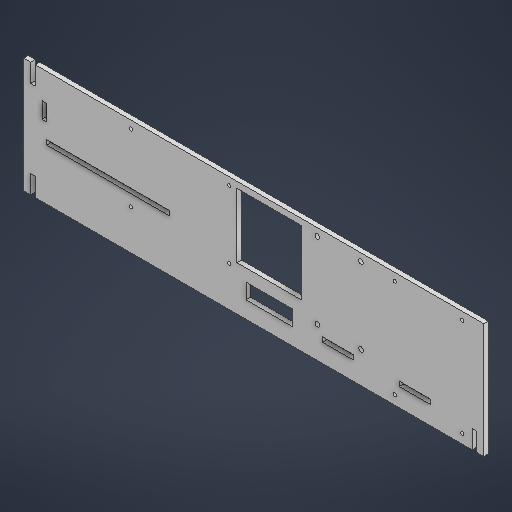
# Autodesk Inventor part: 2ndSideboard
Saved by Autodesk Inventor 2027 (Build 310192000, 192)
## iProperties
Created: 2026-06-01
Part Number: 2ndSideboard
Material: Generic
Document SubType Name: Modeling
Designer: alexy
Density: 1 g/cm^3
Appearance: Default
Author: alexy
Autodesk Inventor part; units mm, degrees
ref_plane "YZ Plane" through (0, 0, 0) normal (1, 0, 0) x (0, 1, 0)
ref_plane "XZ Plane" through (0, 0, 0) normal (0, 1, 0) x (-1, 0, 0)
ref_plane "XY Plane" through (0, 0, 0) normal (0, 0, 1) x (1, 0, 0)
sketch "Sketch1" plane through (0, 0, 0) normal (0, 0, 1) x (1, 0, 0)
  line L0 (0, 0) -> (300, 0)
  line L1 (300, 0) -> (300, 65)
  line L2 (300, 65) -> (0, 65)
  line L3 (0, 65) -> (0, 0)
  line L4 (0, 0) -> (300, 0)
  line L5 (300, 0) -> (300, -10)
  line L6 (300, -10) -> (0, -10)
  line L7 (0, -10) -> (0, 0)
  dimension "d0" = 300
  dimension "d1" = 65
  dimension "d2" = 10
  constraints: 16 end point, 4 parallel, 2 horizontal, 2 perpendicular, 1 vertical alignment
  measures "d0" distance of L1.end L2.end
  measures "d1" distance of L0.end L1.end
  measures "d2" distance of L4.end L5.end
extrude "Extrusion1" add sketch "Sketch1" along normal blind 3
sketch "Sketch3" plane through (0, 0, 3) normal (0, 0, 1) x (1, 0, 0)
  line L0 (139, 61) -> (181, 61)
  line L1 (181, 61) -> (181, 19)
  line L2 (181, 19) -> (139, 19)
  line L3 (139, 19) -> (139, 61)
  line L4 (139, 61) -> (181, 19) construction
  line L5 (181, 61) -> (139, 19) construction
  line L6 (300, -10) -> (300, 65) projected
  line L7 (300, 65) -> (0, 65) projected
  line L8 (0, 65) -> (0, -10) projected
  line L9 (145, 11) -> (175, 11)
  line L10 (175, 11) -> (175, 1)
  line L11 (175, 1) -> (145, 1)
  line L12 (145, 1) -> (145, 11)
  line L13 (145, 11) -> (175, 1) construction
  line L14 (175, 11) -> (145, 1) construction
  point P0 (0, 0)
  point P1 (160, 40)
  point P2 (160, 6)
  dimension "d12" = 25
  dimension "d13" = 42
  dimension "d14" = 42
  dimension "d19" = 160
  dimension "d57" = 8
  dimension "d58" = 30
  dimension "d59" = 10
  constraints: 24 end point, 4 midpoint, 4 parallel, 2 horizontal, 2 perpendicular, 1 vertical alignment
  measures "d12" distance from line of L7 point (160, 40)
  measures "d13" distance of L0.end L1.end
  measures "d14" distance of L1.end L2.end
  measures "d19" distance from line of L8 point (160, 40)
  measures "d57" distance between parallel lines of L2 L9
  measures "d58" distance of L10.end L11.end
  measures "d59" distance of L9.end L10.end
extrude "Extrusion2" cut sketch "Sketch3" against normal blind 3
sketch "Sketch2" plane through (0, 0, 3) normal (0, 0, 1) x (1, 0, 0)
  line L0 (0, -10) -> (300, -10) projected
  line L1 (4.5, -10) -> (7.5, -10)
  line L2 (7.5, -10) -> (7.5, 2)
  line L3 (7.5, 2) -> (4.5, 2)
  line L4 (4.5, 2) -> (4.5, -10)
  line L5 (295.5, -10) -> (292.5, -10)
  line L6 (292.5, -10) -> (292.5, 2)
  line L7 (292.5, 2) -> (295.5, 2)
  line L8 (295.5, 2) -> (295.5, -10)
  line L9 (300, 65) -> (0, 65) projected
  line L10 (4.5, 65) -> (7.5, 65)
  line L11 (7.5, 65) -> (7.5, 53)
  line L12 (7.5, 53) -> (4.5, 53)
  line L13 (4.5, 53) -> (4.5, 65)
  line L14 (0, 65) -> (0, -10) projected
  point P0 (0, 0)
  point P1 (294, 2)
  dimension "d5" = 4.5
  dimension "d6" = 12
  dimension "d7" = 3
  dimension "d8" = 6
  dimension "d9" = 3
  dimension "d53" = 12
  dimension "d54" = 3
  dimension "d55" = 4.5
  constraints: 24 end point, 6 parallel, 3 horizontal, 3 perpendicular, 3 point on line, 1 horizontal alignment, 1 midpoint
  measures "d5" distance of L0.start L1.start
  measures "d6" distance of L1.end L2.end
  measures "d7" distance of L1.start L1.end
  measures "d8" horizontal distance of L0.end point (294, 2)
  measures "d9" distance between parallel lines of L6 L8
  measures "d53" distance of L10.end L11.end
  measures "d54" distance of L11.end L12.end
  measures "d55" distance between parallel lines of L14 L13
extrude "Extrusion3" cut sketch "Sketch2" against normal blind 3
sketch "Sketch4" plane through (0, 0, 3) normal (0, 0, 1) x (1, 0, 0)
  line L0 (15.05, 26.5) -> (95.15, 26.5)
  line L1 (95.15, 26.5) -> (95.15, 23.45)
  line L2 (95.15, 23.45) -> (15.05, 23.45)
  line L3 (15.05, 23.45) -> (15.05, 26.5)
  line L4 (12, 47) -> (15.05, 47)
  line L5 (15.05, 47) -> (15.05, 36.5)
  line L6 (15.05, 36.5) -> (12, 36.5)
  line L7 (12, 36.5) -> (12, 47)
  line L8 (0, 65) -> (0, -10) projected
  point P0 (0, 0)
  point P1 (139, 19)
  dimension "d20" = 80.1
  dimension "d21" = 3.05
  dimension "d22" = 3.05
  dimension "d23" = 10.5
  dimension "d28" = 12
  dimension "d56" = 18
  dimension "d60" = 10
  constraints: 16 end point, 4 parallel, 2 horizontal, 2 perpendicular, 1 vertical alignment
  measures "d20" distance of L1.end L2.end
  measures "d21" distance of L0.end L1.end
  measures "d22" distance of L4.start L4.end
  measures "d23" distance of L6.end L4.start
  measures "d28" distance from line of L8 L4.start
  measures "d56" vertical distance of L8.start L4.start
  measures "d60" distance of L0.start L5.end
extrude "Extrusion4" cut sketch "Sketch4" against normal blind 3
sketch "Sketch5" plane through (0, 0, 3) normal (0, 0, 1) x (1, 0, 0)
  circle A0 centre (191.5, 60) radius 1.55
  circle A1 centre (220, 60) radius 1.55
  circle A2 centre (220, 10.5) radius 1.55
  circle A3 centre (191.5, 10.5) radius 1.55
  line L0 (300, -10) -> (300, 65) projected
  point P0 (0, 0)
  dimension "d31" = 28.5
  dimension "d32" = 49.5
  dimension "d33" = 3.1
  dimension "d34" = 3.1
  dimension "d35" = 3.1
  dimension "d36" = 3.1
  dimension "d37" = 80
  dimension "d38" = 5
  constraints: 4 centre point, 2 horizontal alignment, 2 vertical alignment
  measures "d31" distance of A1.centre A0.centre
  measures "d32" distance of A2.centre A1.centre
  measures "d33" diameter of A0
  measures "d34" diameter of A1
  measures "d35" diameter of A2
  measures "d36" diameter of A3
  measures "d37" distance from line of L0 A1.centre
  measures "d38" vertical distance of L0.end A1.centre
extrude "Extrusion5" cut sketch "Sketch5" against normal blind 3
sketch "Sketch6" plane through (0, 0, 3) normal (0, 0, 1) x (1, 0, 0)
  circle A0 centre (242, 60) radius 1.1
  circle A1 centre (286, 60) radius 1.1
  circle A2 centre (286, -4) radius 1.1
  circle A3 centre (242, -4) radius 1.1
  circle A4 centre (220, 60) radius 1.55 projected
  circle A5 centre (70, 60) radius 1.1
  circle A6 centre (134, 60) radius 1.1
  circle A7 centre (134, 16) radius 1.1
  circle A8 centre (70, 16) radius 1.1
  point P0 (0, 0)
  point P1 (300, 65)
  point P2 (0, 65)
  dimension "d41" = 2.2
  dimension "d42" = 2.2
  dimension "d43" = 2.2
  dimension "d44" = 2.2
  dimension "d45" = 64
  dimension "d46" = 44
  dimension "d50" = 5
  dimension "d51" = 14
  dimension "d61" = 64
  dimension "d62" = 44
  dimension "d63" = 2.2
  dimension "d64" = 2.2
  dimension "d65" = 2.2
  dimension "d66" = 2.2
  dimension "d67" = 70
  dimension "d68" = 5
  constraints: 8 centre point, 4 horizontal alignment, 4 vertical alignment
  measures "d41" diameter of A0
  measures "d42" diameter of A1
  measures "d43" diameter of A2
  measures "d44" diameter of A3
  measures "d45" distance of A3.centre A0.centre
  measures "d46" distance of A0.centre A1.centre
  measures "d50" vertical distance of point (300, 65) A1.centre
  measures "d51" horizontal distance of point (300, 65) A1.centre
  measures "d61" distance of A5.centre A6.centre
  measures "d62" distance of A7.centre A6.centre
  measures "d63" diameter of A6
  measures "d64" diameter of A7
  measures "d65" diameter of A8
  measures "d66" diameter of A5
  measures "d67" horizontal distance of point (0, 65) A5.centre
  measures "d68" vertical distance of point (0, 65) A5.centre
extrude "Extrusion6" cut sketch "Sketch6" against normal blind 3 contours A0 | A1 | A2 | A3 | A5 | A6 | A7 | A8
sketch "Sketch7" plane through (0, 0, 3) normal (0, 0, 1) x (1, 0, 0)
  line L0 (244.95, 5.05) -> (265, 5.05)
  line L1 (265, 5.05) -> (265, 2)
  line L2 (265, 2) -> (244.95, 2)
  line L3 (244.95, 2) -> (244.95, 5.05)
  line L4 (194.9, 5.05) -> (215, 5.05)
  line L5 (215, 5.05) -> (215, 2)
  line L6 (215, 2) -> (194.9, 2)
  line L7 (194.9, 2) -> (194.9, 5.05)
  line L8 (300, -10) -> (300, 65) projected
  point P0 (0, 0)
  dimension "d69" = 20.05
  dimension "d70" = 3.05
  dimension "d73" = 20.1
  dimension "d74" = 29.95
  dimension "d75" = 35
  dimension "d76" = 12
  constraints: 16 end point, 4 parallel, 2 horizontal, 2 horizontal alignment, 2 perpendicular
  measures "d69" distance of L1.end L2.end
  measures "d70" distance of L0.end L1.end
  measures "d73" distance of L5.end L6.end
  measures "d74" distance of L2.end L5.end
  measures "d75" distance from line of L8 L1.end
  measures "d76" vertical distance of L8.start L1.end
extrude "Extrusion7" cut sketch "Sketch7" against normal blind 3
body "Solid1"
